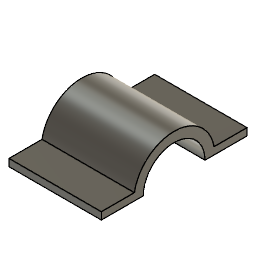
TopLegClamp (Autodesk Fusion 360 design; units mm, degrees)
Autodesk Fusion 360 part; units mm, degrees
sketch "Sketch1" plane through (0, 0, 0) normal (1, 0, 0) x (0, 1, 0)
  line L0 (-116.8301, 0) -> (116.8301, 0) construction
  arc A0 (12.7, 0) -> (-12.7, 0) centre (0, 0) ccw
  arc A1 (16.4283, 3) -> (-16.4283, 3) centre (0, 0) ccw
  line L1 (-12.7, 0) -> (-30.05, 0)
  line L2 (-30.05, 0) -> (-30.05, 3)
  line L3 (-30.05, 3) -> (-16.4283, 3)
  line L4 (0, 0) -> (0, 21) construction
  line L5 (30.05, 3) -> (16.4283, 3)
  line L6 (30.05, 0) -> (30.05, 3)
  line L7 (12.7, 0) -> (30.05, 0)
  dimension "d1" = 12.7
  dimension "d2" = 4
  dimension "d3" = 30.05
  dimension "d4" = 3
  constraint midpoint L0 A0.centre
  constraint coincident A0.centre A1.centre
  constraint horizontal L0
  constraint coincident L0 A0.start
  constraint coincident L0 A0.end
  constraint coincident L0 L1.end
  constraint perpendicular L1 L2
  constraint perpendicular L2 L3
  constraint coincident A1.end L3.end
  constraint perpendicular L0 L4
  constraint symmetric A0.end L4 A0.start
  constraint symmetric L1.end L4 L6.start
  constraint symmetric L2.end L4 L5.start
  constraint symmetric A1.end L4 A1.start
  measures "d1" radius of A0
  measures "d3" distance of A0.centre L1.end
  measures "d4" distance of L1.end L2.end
extrude "Extrude1" add sketch "Sketch1" along normal mid plane 38.1
equation "d1 = 1 in / 2"
equation "d3 = 60.1 mm / 2"
